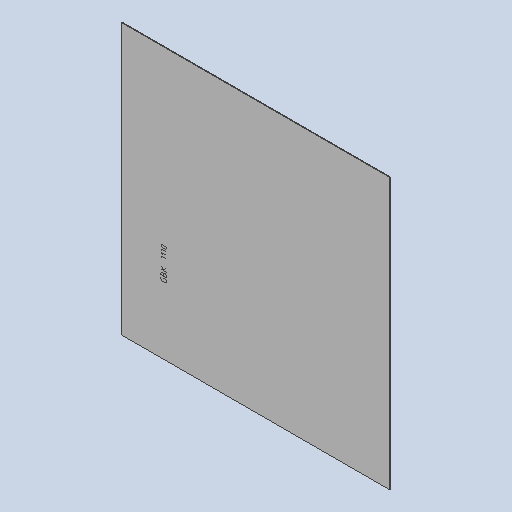
# Autodesk Inventor part: GBK 2111 shield 1
Saved by Autodesk Inventor 2026 (Build 300175000, 175)
## iProperties
Created: 2026-04-17
Part Number: GBK 2111 shield 1
Material: Steel
Document SubType Name: Sheet Metal
Designer: pokla
Stock Number: 1111
Mass: 69243.3 g
Surface Area: 44341.6 cm^2
Volume: 8820.8 cm^3
Density: 7.85 g/cm^3
Flat Pattern Width: 148 cm
Flat Pattern Length: 149 cm
Flat Pattern Area: 22052 cm^2
Sheet Metal Rule: По умолчанию_мм
Sheet Metal Width: 1480,000 mm
Sheet Metal Length: 1490,000 mm
Sheet Metal Area: 2205200,000 mm^2
Appearance: Default
Author: admin
Autodesk Inventor part; units mm, degrees
ref_plane "YZ Plane" through (0, 0, 0) normal (1, 0, 0) x (0, 1, 0)
ref_plane "XZ Plane" through (0, 0, 0) normal (0, 1, 0) x (-1, 0, 0)
ref_plane "XY Plane" through (0, 0, 0) normal (0, 0, 1) x (1, 0, 0)
sketch "Sketch1" plane through (0, 0, 0) normal (0, 0, 1) x (1, 0, 0)
  line L0 (740, -745) -> (-740, -745)
  line L1 (-740, -745) -> (-740, 745)
  line L2 (-740, 745) -> (740, 745)
  line L3 (740, 745) -> (740, -745)
  line L4 (740, -745) -> (-740, 745) construction
  line L5 (-740, -745) -> (740, 745) construction
  point P0 (0, 0)
  dimension "d0" = 1480
  dimension "d1" = 1490
  measures "d0" distance of L1.end L2.end
  measures "d1" distance of L0.end L1.end
extrude "Plate1" add sketch "Sketch1" along normal blind 4
sketch "Sketch2" plane through (0, 0, 4) normal (0, 0, 1) x (1, 0, 0)
  line L0 (-522.6585, -376.8166) -> (-522.6585, 27.0801) construction
  line L1 (-522.6585, 27.0801) -> (-472.0358, 27.0801) construction
  line L2 (-472.0358, 27.0801) -> (-472.0358, -376.8166) construction
  line L3 (-472.0358, -376.8166) -> (-522.6585, -376.8166) construction
  point P0 (0, 0)
  constraints: 2 other
mark "Mark1"
equation "\"d0\" = Лист_ширина"
equation "\"d1\" = 0.5 * Лист_длина"
equation "\"d2\" = Thickness"
equation "\"BendRadius\" = Thickness"
equation "\"BendReliefWidth\" = Thickness"
equation "\"BendReliefDepth\" = 0.5 * Thickness"
equation "\"CornerReliefSize\" = 4 * Thickness"
equation "\"MinimumRemnant\" = 2 * Thickness"
equation "\"TransitionRadius\" = BendRadius"
equation "\"JacobiRadiusSize\" = BendRadius"
equation "\"GapSize\" = Thickness"
equation "\"Лист_ширина\" = 1480"
equation "\"Лист_длина\" = 2980"
equation "\"Thickness\" = 4"
body "Solid1"
